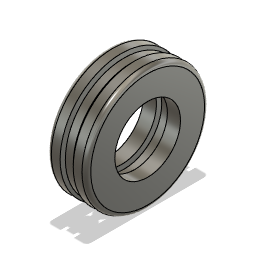
Bearing_GOST_23526-79_9000 (Autodesk Fusion 360 design; units mm, degrees)
Autodesk Fusion 360 part; units mm, degrees
sketch "Sketch1" plane through (0, 0, 0) normal (0, 0, 1) x (1, 0, 0)
  line L0 (-79.6992, 0) -> (79.6992, 0)
  line L1 (-4.5, 14) -> (-1.5, 14)
  line L2 (-1.5, 14) -> (-1.5, 8)
  line L3 (-1.5, 8) -> (-4.5, 8)
  line L4 (-4.5, 8) -> (-4.5, 14)
  line L5 (1.5, 14) -> (4.5, 14)
  line L6 (4.5, 14) -> (4.5, 7.5)
  line L7 (4.5, 7.5) -> (1.5, 7.5)
  line L8 (1.5, 7.5) -> (1.5, 14)
  line L9 (-1.5, 12.5) -> (1.5, 12.5)
  line L10 (1.5, 12.5) -> (1.5, 9.5)
  line L11 (1.5, 9.5) -> (-1.5, 9.5)
  line L12 (-1.5, 9.5) -> (-1.5, 12.5)
  line L13 (-0.9, 13.4) -> (0.9, 13.4)
  line L14 (0.9, 13.4) -> (0.9, 8.6)
  line L15 (0.9, 8.6) -> (-0.9, 8.6)
  line L16 (-0.9, 8.6) -> (-0.9, 13.4)
  line L17 (0, 13.4) -> (0, 8.6)
  point P0 (-1.5, 11)
  point P1 (-1.5, 11)
  point P2 (0, 12.5)
  point P3 (0, 11)
  dimension "d1" = 9
  dimension "d2" = 15
  dimension "d3" = 16
  dimension "d4" = 28
  dimension "d5" = 28
  dimension "d6" = 1.8
  dimension "d7" = 4.8
  dimension "d8" = 3
  dimension "d9" = 3
  constraint horizontal L0
  constraint midpoint L0 origin
  constraint horizontal L1
  constraint vertical L2
  constraint horizontal L3
  constraint vertical L4
  constraint horizontal L5
  constraint vertical L6
  constraint horizontal L7
  constraint vertical L8
  constraint horizontal L9
  constraint vertical L10
  constraint horizontal L11
  constraint vertical L12
  constraint coincident L8 L10.end
  constraint coincident L2 L9.start
  constraint horizontal L13
  constraint vertical L14
  constraint horizontal L15
  constraint vertical L16
  constraint midpoint L13 L17.start
  constraint midpoint L15 L17.end
  constraint vertical origin L17.end
  constraint equal L1 L5
  constraint midpoint L2 P1
  constraint midpoint L12 P1
  constraint coincident P1 P0
  constraint midpoint L9 P2
  constraint coincident L17 P2
  constraint midpoint L17 P3
  constraint horizontal P1 P3
  measures "d1" distance of L4 L6
  measures "d6" distance of L13.start L13.end
  measures "d7" distance of L13.start L15.end
  measures "d8" distance of L9 L11
  measures "d9" distance of L5.start L5.end
revolve "Revolve1" add sketch "Sketch1" angle 360 about axis through (-79.6992, 0, 0) along (1, 0, 0) contours L1 L2 L3 L4 L12 | L5 L6 L7 L8 L10 makes body 1 at (-4.5, 11.9479, -0.6955) makes body 2 at (1.5, 11.7812, -0.6955)
revolve "Revolve2" add sketch "Sketch1" angle 360 about axis through (0, 13.4, 0) along (0, -1, 0) separate body contours L2 L9 L11 L12 L16 | L9 L11 L16 L17 makes body 3
revolve "Revolve3" add sketch "Sketch1" angle 360 about axis through (-79.6992, 0, 0) along (1, 0, 0) separate body contours L9 L13 L16 L17 | L9 L11 L16 L17 | L11 L15 L16 L17 | L9 L13 L14 L17 | L9 L11 L14 L17 | L11 L14 L15 L17 makes body 4
pattern_circular "C-Pattern1" count 12 over 360 about axis through (1.75, 0, 0) along (1, 0, 0) of bodies 3 makes body 5 at (-1.4925, 9.0186, 5.3793) makes body 6 at (-1.4925, 5.1207, 9.1679) makes body 7 at (-1.4925, -0.1494, 10.5) makes body 8 at (-1.4925, -5.3793, 9.0186) makes body 9 at (-1.4981, -9.9967, 5.6852) makes body 10 at (-1.4925, -10.5, -0.1494) makes body 11 at (-1.4981, -9.9219, -5.8148) makes body 12 at (-1.4925, -5.1207, -9.1679) makes body 13 at (-1.4925, 0.1494, -10.5) makes body 14 at (-1.4981, 5.8148, -9.9219) makes body 15 at (-1.4925, 9.1679, -5.1207)
fillet "Fillet1" radius 1 2 edges at (-4.5, -5.0626, 13.0526) (4.5, -5.0626, 13.0526) on bodies 1 2
